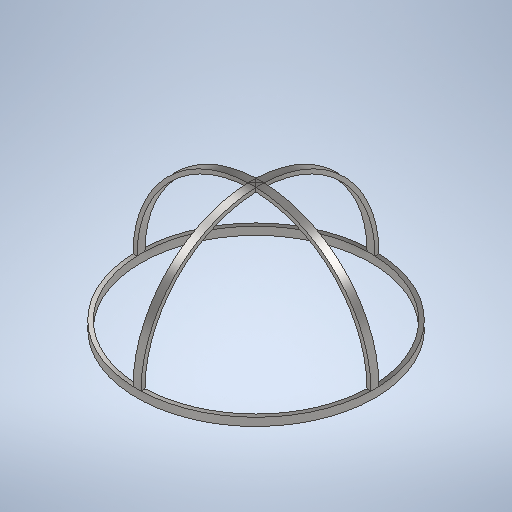
# Autodesk Inventor part: Dome
Saved by Autodesk Inventor 2025.1 (Build 291241000, 241)
## iProperties
Created: 2024-11-07
Part Number: Dome
Material: Steel, Mild
Document SubType Name: Modeling
Designer: smonowar1008
Density: 7.85 g/cm^3
Appearance: Semi-Polished
Author: smonowar1008
Autodesk Inventor part; units mm, degrees
ref_plane "YZ Plane" through (0, 0, 0) normal (1, 0, 0) x (0, 1, 0)
ref_plane "XZ Plane" through (0, 0, 0) normal (0, 1, 0) x (-1, 0, 0)
ref_plane "XY Plane" through (0, 0, 0) normal (0, 0, 1) x (1, 0, 0)
sketch "Sketch1" plane through (0, 0, 0) normal (0, 1, 0) x (-1, 0, 0)
  circle A0 centre (0, 0) radius 95
  circle A1 centre (0, 0) radius 91.825
  dimension "d0" = 190
  dimension "d1" = 183.65
  constraints: 2 centre point, 2 coincident
  measures "d0" diameter of A0
  measures "d1" diameter of A1
extrude "Extrusion1" add sketch "Sketch1" along normal blind 6.35
sketch "Sketch2" plane through (0, 0, 0) normal (1, 0, 0) x (0, 1, 0)
  line L0 (6.35, -95) -> (6.35, 95) projected
  arc A0 (101.35, 0) -> (6.35, 95) centre (6.35, 0) ccw
  arc A1 (98.175, 0) -> (6.35, 91.825) centre (6.35, 0) ccw
  line L1 (101.35, 0) -> (98.175, 0)
  line L2 (6.35, 95) -> (6.35, 91.825)
  point P0 (0, 0)
  dimension "d11" = 91.825
  constraints: 4 end point, 4 point on circle, 2 centre point, 1 coincident, 1 collinear, 1 horizontal, 1 midpoint, 1 point on line
  measures "d11" radius of A1
extrude "Curved Bar 1" add sketch "Sketch2" along normal mid plane 6.35
sketch "Sketch4" plane through (0, 0, 0) normal (1, 0, 0) x (0, 1, 0)
  line L0 (6.35, -95) -> (6.35, 95) projected
  arc A0 (6.35, -95) -> (101.35, 0) centre (6.35, 0) ccw
  arc A1 (6.35, -91.825) -> (98.175, 0) centre (6.35, 0) ccw
  line L1 (101.35, 0) -> (98.175, 0)
  line L2 (6.35, -95) -> (6.35, -91.825)
  point P0 (0, 0)
  point P1 (6.35, 94.9469)
  dimension "d18" = 91.825
  constraints: 4 end point, 4 point on circle, 2 centre point, 1 coincident, 1 horizontal, 1 midpoint, 1 perpendicular
  measures "d18" radius of A1
extrude "Extrusion4" add sketch "Sketch4" along normal mid plane 6.35
sketch "Sketch5" plane through (0, 0, 0) normal (0, 0, 1) x (1, 0, 0)
  line L0 (0, 6.35) -> (-3.175, 6.35) projected
  line L1 (-3.175, 101.35) -> (3.175, 101.35) projected
  line L2 (-3.175, 6.35) -> (-95, 6.35) projected
  arc A0 (0, 101.35) -> (-95, 6.35) centre (0, 6.35) ccw
  arc A1 (0, 98.175) -> (-91.825, 6.35) centre (0, 6.35) ccw
  line L3 (0, 101.35) -> (0, 98.175)
  line L4 (-91.825, 6.35) -> (-95, 6.35)
  point P0 (0, 0)
  point P1 (-91.825, 6.35)
  dimension "d21" = 91.825
  constraints: 4 end point, 4 point on circle, 2 centre point, 1 coincident, 1 midpoint, 1 perpendicular, 1 vertical
  measures "d21" radius of A1
extrude "Extrusion5" add sketch "Sketch5" along normal mid plane 6.35
sketch "Sketch6" plane through (0, 0, 0) normal (0, 0, 1) x (1, 0, 0)
  line L0 (0, 6.35) -> (-3.175, 6.35) projected
  line L1 (95, 6.35) -> (3.175, 6.35) projected
  line L2 (0, 101.2969) -> (0, 101.35) projected
  arc A0 (95, 6.35) -> (0, 101.35) centre (0, 6.35) ccw
  line L3 (0, 6.35) -> (91.825, 6.35) projected
  arc A1 (91.825, 6.35) -> (0, 98.175) centre (0, 6.35) ccw
  line L4 (95, 6.35) -> (91.825, 6.35)
  line L5 (0, 101.35) -> (0, 98.175)
  point P0 (0, 0)
  dimension "d24" = 91.825
  constraints: 5 point on circle, 4 end point, 2 centre point, 1 coincident, 1 horizontal, 1 perpendicular, 1 point on line
  measures "d24" radius of A1
extrude "Extrusion6" add sketch "Sketch6" along normal mid plane 6.35
body "Solid1"
